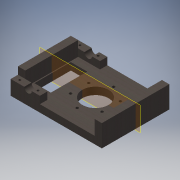
# Autodesk Inventor part: SupportForAxel
Saved by Autodesk Inventor 2019.3 (Build 233278000, 278)
## iProperties
Created: 2019-01-06
Part Number: SupportForAxel
Material: PBT Plastic
Document SubType Name: Modeling
Designer: steele
Density: 1.31 g/cm^3
Appearance: Walnut
Author: steele
Autodesk Inventor part; units mm, degrees
ref_plane "YZ Plane" through (0, 0, 0) normal (1, 0, 0) x (0, 1, 0)
ref_plane "XZ Plane" through (0, 0, 0) normal (0, 1, 0) x (-1, 0, 0)
sketch "Sketch10" plane through (0, 0, 0) normal (0, 1, 0) x (-1, 0, 0)
  line L0 (88.9, 58.7375) -> (-88.9, 58.7375)
  line L1 (-88.9, 58.7375) -> (-88.9, -58.7375)
  line L2 (-88.9, -58.7375) -> (88.9, -58.7375)
  line L3 (88.9, -58.7375) -> (88.9, 58.7375)
  line L4 (88.9, 58.7375) -> (-88.9, -58.7375) construction
  line L5 (-88.9, 58.7375) -> (88.9, -58.7375) construction
  circle A0 centre (0, 0) radius 22.86
  dimension "d56" = 177.8
  dimension "d57" = 45.72
  constraints: 12 end point, 2 midpoint, 2 parallel, 1 centre point, 1 coincident, 1 horizontal, 1 perpendicular
  measures "d56" distance of L0.start L0.end
  measures "d57" diameter of A0
extrude "Extrusion5" add sketch "Sketch10" against normal blind 12.7
sketch "Sketch11" plane through (0, 0, 0) normal (0, 1, 0) x (1, 0, 0)
  point P0 (0, 0)
  point P1 (0, 31.75)
  dimension "d60" = 31.75
  measures "d60" distance of point (0, 31.75) point (0, 0)
hole "Hole4" at (0, 0, -31.75) direction (0, -1, 0) diameter 2.6416 end through all counterbore diameter 4.699 counterbore depth 7.1374 thread size "6-32 UNC" class "2B" standard "ANSI Unified Screw Threads"
pattern_circular "Circular Pattern1" count 6 over 360 about axis through (0, -10, 0) along (0, 1, 0) of "Hole4"
sketch "Sketch12" plane through (0, 0, 0) normal (0, 1, 0) x (1, 0, 0)
  line L0 (-88.9, -58.7375) -> (-88.9, 58.7375) projected
  line L1 (-88.9, 58.7375) -> (-38.1, 58.7375)
  line L2 (-38.1, 58.7375) -> (-38.1, 46.0375)
  line L3 (-38.1, 46.0375) -> (-88.9, 46.0375)
  line L4 (-88.9, 46.0375) -> (-88.9, 58.7375)
  point P0 (0, 0)
  dimension "d71" = 12.7
  dimension "d72" = 50.8
  constraints: 8 end point, 2 parallel, 1 horizontal, 1 perpendicular
  measures "d71" distance between parallel lines of L3 L1
  measures "d72" distance of L2.end L3.end
extrude "Extrusion6" add sketch "Sketch12" along normal blind 12.7
mirror "Mirror2" about plane through (0, 0, 0) normal (0, 0, 1) of "Extrusion6"
sketch "Sketch13" plane through (88.9, -12.7, -58.7375) normal (0, 0, -1) x (-1, 0, 0)
  line L0 (127, 25.4) -> (177.8, 25.4) projected
  circle A0 centre (147.6375, 25.4) radius 6.604
  point P0 (88.9, 12.7)
  dimension "d75" = 13.208
  constraints: 1 centre point, 1 point on line
  measures "d75" diameter of A0
extrude "Extrusion7" cut sketch "Sketch13" against normal through all
sketch "Sketch14" plane through (0, 0, 0) normal (0, 1, 0) x (1, 0, 0)
  line L0 (-88.9, 46.0375) -> (-76.2, 46.0375)
  line L1 (-76.2, 46.0375) -> (-76.2, -46.0375)
  line L2 (-76.2, -46.0375) -> (-88.9, -46.0375)
  line L3 (-88.9, -46.0375) -> (-88.9, 46.0375)
  point P0 (0, 0)
  dimension "d78" = 12.7
  constraints: 8 end point, 2 parallel, 1 horizontal, 1 perpendicular
  measures "d78" distance between parallel lines of L1 L3
extrude "Extrusion8" add sketch "Sketch14" along normal blind 25.4
sketch "Sketch15" plane through (0, 0, 0) normal (0, 1, 0) x (1, 0, 0)
  line L0 (88.9, 58.7375) -> (-38.1, 58.7375) projected
  line L1 (-38.1, -58.7375) -> (88.9, -58.7375) projected
  line L2 (57.15, 58.7375) -> (69.85, 58.7375)
  line L3 (69.85, 58.7375) -> (69.85, -58.7375)
  line L4 (69.85, -58.7375) -> (57.15, -58.7375)
  line L5 (57.15, -58.7375) -> (57.15, 58.7375)
  line L6 (-88.9, 46.0375) -> (-88.9, -46.0375) projected
  point P0 (0, 0)
  dimension "d81" = 12.7
  dimension "d82" = 146.05
  constraints: 8 end point, 2 parallel, 2 point on line, 1 horizontal, 1 perpendicular
  measures "d81" distance between parallel lines of L3 L5
  measures "d82" distance between parallel lines of L5 L6
extrude "Extrusion9" add sketch "Sketch15" along normal blind 25.4
sketch "Sketch16" plane through (0, 0, 0) normal (0, 1, 0) x (1, 0, 0)
  line L0 (88.9, 58.7375) -> (69.85, 58.7375) projected
  line L1 (88.9, -58.7375) -> (69.85, -58.7375)
  line L2 (69.85, -58.7375) -> (69.85, 58.7375)
  line L3 (69.85, 58.7375) -> (88.9, 58.7375)
  line L4 (88.9, 58.7375) -> (88.9, -58.7375)
  point P0 (0, 0)
  constraints: 8 end point, 2 parallel, 1 horizontal, 1 perpendicular
extrude "Extrusion10" cut sketch "Sketch16" against normal through all
sketch "Sketch18" plane through (0, -12.7, 0) normal (0, -1, 0) x (1, 0, 0)
  line L0 (-88.9, 58.7375) -> (-88.9, 46.0375) construction
  line L1 (-88.9, 52.3875) -> (69.85, 52.3875) construction
  line L2 (69.85, 58.7375) -> (69.85, -58.7375) construction
  line L3 (-88.9, -58.7375) -> (-88.9, -46.0375) construction
  line L4 (-88.9, -52.3875) -> (69.85, -52.3875) construction
  line L5 (-65.3415, -46.0375) -> (-65.3415, -58.7375) projected
  line L6 (-65.3415, -58.7375) -> (-88.9, -58.7375) projected
  line L7 (-88.9, -58.7375) -> (-88.9, -46.0375) projected
  line L8 (-88.9, -46.0375) -> (-76.2, -46.0375) projected
  line L9 (-76.2, -46.0375) -> (-65.3415, -46.0375) projected
  line L10 (-52.1335, -58.7375) -> (-52.1335, -46.0375) projected
  line L11 (-52.1335, -46.0375) -> (-38.1, -46.0375) projected
  line L12 (-38.1, -46.0375) -> (-38.1, -58.7375) projected
  line L13 (-38.1, -58.7375) -> (-52.1335, -58.7375) projected
  line L14 (-88.9, 58.7375) -> (-88.9, -58.7375) projected
  line L15 (-88.9, 0) -> (69.85, 0) construction
  line L16 (69.85, -58.7375) -> (69.85, 58.7375) construction
  point P0 (0, 0)
  point P1 (-79.375, -52.3875)
  point P2 (-47.625, -52.3875)
  point P3 (-79.375, 52.3875)
  point P4 (-47.625, 52.3875)
  dimension "d94" = 9.525
  dimension "d95" = 9.525
  constraints: 6 end point, 4 point on line, 3 midpoint, 2 symmetric about line, 1 horizontal, 1 perpendicular, 2 other
  measures "d95" distance from line of point (-47.625, -52.387) L12
hole "Hole6" at (-79.375, -12.7, -52.3875) at (-47.625, -12.7, -52.3875) at (-79.375, -12.7, 52.3875) at (-47.625, -12.7, 52.3875) direction (0, 1, 0) diameter 3.81 end through all clearance for "Flat Head Machine Screw (82)" size "#6" standard "Ansi Unified Screw Threads"
sketch "Sketch19" plane through (0, 0, 0) normal (0, 1, 0) x (1, 0, 0)
  line L0 (-74.6125, 31.75) -> (-74.6125, -31.75)
  line L1 (-74.6125, -31.75) -> (-46.0375, -31.75)
  line L2 (-46.0375, -31.75) -> (-46.0375, 31.75)
  line L3 (-46.0375, 31.75) -> (-74.6125, 31.75)
  line L4 (-74.6125, 31.75) -> (-46.0375, -31.75) construction
  line L5 (-74.6125, -31.75) -> (-46.0375, 31.75) construction
  point P0 (0, 0)
  point P1 (-60.325, 0)
  constraints: 12 end point, 2 midpoint, 2 parallel, 1 perpendicular, 1 vertical
extrude "Extrusion11" cut sketch "Sketch19" against normal blind 12.7
equation "\"length\" = 69.0372"
body "Solid2"
